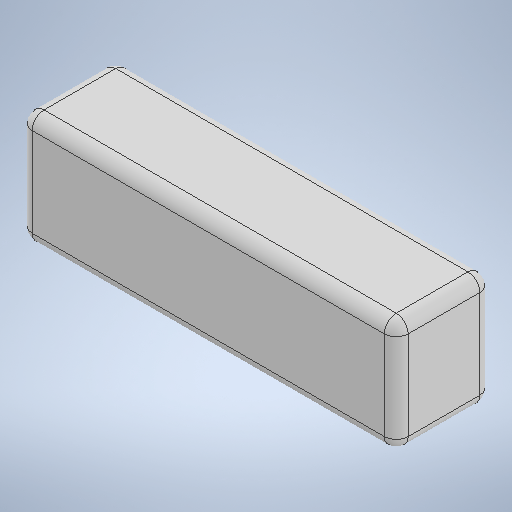
# Autodesk Inventor part: usbhubnewblockboostermount
Saved by Autodesk Inventor 2025.1 (Build 291241000, 241)
## iProperties
Created: 2024-10-26
Part Number: usbhubnewblockboostermount
Material: Generic
Document SubType Name: Modeling
Designer: ishaa
Density: 1 g/cm^3
Appearance: Default
Author: ishaa
Autodesk Inventor part; units mm, degrees
ref_plane "YZ Plane" through (0, 0, 0) normal (1, 0, 0) x (0, 1, 0)
ref_plane "XZ Plane" through (0, 0, 0) normal (0, 1, 0) x (-1, 0, 0)
ref_plane "XY Plane" through (0, 0, 0) normal (0, 0, 1) x (1, 0, 0)
sketch "Sketch1" plane through (0, 0, 0) normal (0, 0, 1) x (1, 0, 0)
  line L0 (-50, -15) -> (50, -15)
  line L1 (50, -15) -> (50, 15)
  line L2 (50, 15) -> (-50, 15)
  line L3 (-50, 15) -> (-50, -15)
  line L4 (-50, -15) -> (50, 15) construction
  line L5 (50, -15) -> (-50, 15) construction
  point P0 (0, 0)
  dimension "d0" = 100
  dimension "d1" = 30
  constraints: 12 end point, 2 midpoint, 2 parallel, 1 horizontal, 1 perpendicular
  measures "d0" distance of L2.end L1.end
  measures "d1" distance of L1.end L0.end
extrude "Extrusion1" add sketch "Sketch1" along normal blind 25.4
fillet "Fillet1" radius 3.175 12 edges at (50, 0, 25.4) (50, 0, 0) (50, 15, 12.7) (0, 15, 25.4) (0, 15, 0) (-50, 15, 12.7) (-50, 0, 25.4) (-50, 0, 0) (-50, -15, 12.7) (0, -15, 25.4) (50, -15, 12.7) (0, -15, 0)
body "Solid1"
